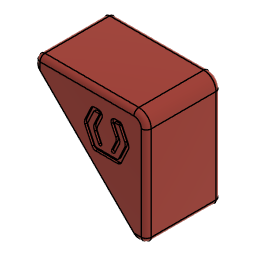
LogoRahmen (Autodesk Fusion 360 design; units mm, degrees)
Autodesk Fusion 360 part; units mm, degrees
box "Grundkörper Quader1" add length 240 width 240 height 3.2 placed x (0, 0, 1) y (1, 0, 0) z (0, 1, 0) at (0, 0, 0) makes body 1 in component "Canvas"
sketch "Skizze10" plane through (0, 0, 0) normal (0, -1, 0) x (1, 0, 0)
  line L0 (240, 240) -> (0, 240)
  line L1 (0, 240) -> (0, 0)
  line L2 (0, 0) -> (240, 0)
  line L3 (240, 0) -> (240, 240)
  line L4 (240, 0) -> (240, 240)
  line L5 (240, -11) -> (0, -11)
  line L6 (0, -11) -> (0, 8)
  line L7 (0, 8) -> (240, 8)
  line L8 (240, 8) -> (240, -11)
  line L9 (240, 120) -> (0, 120) construction
  line L10 (120, 240) -> (120, 0) construction
  line L11 (0, 251) -> (0, 232)
  line L12 (240, 251) -> (0, 251)
  line L13 (240, 232) -> (240, 251)
  line L14 (0, 232) -> (240, 232)
  line L15 (8, 232) -> (-11, 232)
  line L16 (-11, 232) -> (-11, 8)
  line L17 (-11, 8) -> (8, 8)
  line L18 (8, 8) -> (8, 232)
  line L19 (232, 8) -> (232, 232)
  line L20 (251, 232) -> (251, 8)
  line L21 (251, 8) -> (232, 8)
  line L22 (232, 232) -> (251, 232)
  dimension "d100" = 19
  dimension "d101" = 8
  dimension "d102" = 19
  dimension "d103" = 8
  constraint horizontal L5
  constraint vertical L6
  constraint horizontal L7
  constraint vertical L8
  constraint coincident L1 L6.end
  constraint collinear L4 L8
  constraint midpoint L3 L9.start
  constraint midpoint L1 L9.end
  constraint midpoint L0 L10.start
  constraint midpoint L2 L10.end
  constraint symmetric L5.start L9 L12.start
  constraint symmetric L5.end L9 L11.start
  constraint symmetric L6.end L9 L11.end
  constraint symmetric L7.end L9 L13.start
  constraint horizontal L15
  constraint vertical L16
  constraint horizontal L17
  constraint vertical L18
  constraint collinear L7 L17
  constraint collinear L14 L15
  constraint symmetric L10 L15.start L19.end
  constraint symmetric L10 L15.end L20.start
  constraint symmetric L10 L16.end L20.end
  constraint symmetric L10 L17.end L19.start
  measures "d100" distance of L5 L7
  measures "d101" distance of L2 L7
  measures "d102" distance of L16 L18
  measures "d103" distance of L1 L18
sketch "Skizze11" plane through (0, 3.2, 0) normal (0, 1, 0) x (-1, 0, 0)
  line L0 (0, 240) -> (-240, 240)
  line L1 (-240, 240) -> (-240, 0)
  line L2 (-240, 0) -> (0, 0)
  line L3 (0, 0) -> (0, 240)
  line L4 (-254, 254) -> (-209, 254)
  line L5 (-209, 254) -> (-209, 209)
  line L6 (-209, 209) -> (-254, 209)
  line L7 (-254, 209) -> (-254, 254)
  line L8 (-240, 251) -> (0, 251)
  line L9 (-251, 232) -> (-251, 8)
  line L10 (-209, 251) -> (-240, 251)
  line L11 (-251, 232) -> (-251, 209)
  line L12 (-251, 232) -> (-240, 232)
  line L13 (-240, 232) -> (-240, 251)
  line L14 (-240, 240) -> (-209, 240)
  line L15 (-240, 232) -> (-240, 209)
  dimension "d104" = 3
  dimension "d105" = 3
  dimension "d106" = 45
  dimension "d107" = 45
  constraint horizontal L4
  constraint vertical L5
  constraint horizontal L6
  constraint vertical L7
  constraint coincident L5 L10.start
  constraint coincident L8 L10.start
  constraint coincident L8.start L10.end
  constraint coincident L9.start L11.start
  constraint coincident L6 L11.end
  constraint coincident L9 L11.end
  constraint coincident L1 L12.end
  constraint perpendicular L1 L12
  constraint coincident L0.end L1.start
  constraint coincident L5 L14.end
  constraint coincident L0 L14.end
  constraint coincident L6 L15.end
  constraint coincident L1 L15.end
  measures "d104" distance of L4 L8
  measures "d105" distance of L7 L9
  measures "d106" distance of L5 L7
  measures "d107" distance of L4 L6
extrude "Extrusion1" add sketch "Skizze10" along normal blind 5 separate body contours L0 L1 L3 L4 L11 L13 L14 L15 L22 | L0 L11 L12 L13 makes body 2 in component "Rahmen"
extrude "Extrusion2" add sketch "Skizze10" along normal blind 5 separate body contours L3 L4 L20 L21 L22 | L3 L4 L7 L14 L19 L21 L22 makes body 3 in component "Rahmen"
extrude "Extrusion3" add sketch "Skizze10" along normal blind 5 separate body contours L1 L2 L3 L4 L6 L7 L8 L17 L21 | L2 L5 L6 L8 makes body 4 in component "Rahmen"
extrude "Extrusion4" add sketch "Skizze10" along normal blind 5 separate body contours L1 L7 L14 L15 L17 L18 | L1 L15 L16 L17 makes body 5 in component "Rahmen"
extrude "Extrusion1'" add sketch "Skizze11" along normal blind 27 from surface at -8 separate body contours L1 L4 L5 L6 L7 L8 L9 L10 L11 L12 L13 makes body 6 in component "Ecke"
sketch "Skizze1" plane through (0, -4.8, 0) normal (0, -1, 0) x (1, 0, 0) in component "Ecke"
  line L0 (240, 232) -> (251, 232)
  line L1 (251, 232) -> (251, 209)
  line L2 (251, 209) -> (254, 209)
  line L3 (254, 209) -> (254, 254)
  line L4 (254, 254) -> (209, 254)
  line L5 (209, 254) -> (209, 251)
  line L6 (209, 251) -> (240, 251)
  line L7 (240, 251) -> (240, 232)
  line L8 (251, 209) -> (209, 251)
  line L9 (209, 254) -> (254, 254)
  line L10 (254, 209) -> (254, 254)
  line L11 (251, 209) -> (254, 209)
  line L12 (209, 251) -> (209, 254)
  constraint coincident L1.end L2.start
  constraint coincident L5.end L6.start
  constraint coincident L4.end L5.start
  constraint coincident L3.end L4.start
  constraint coincident L2.end L3.start
extrude "Extrusion2'" add sketch "Skizze1" along normal blind 3.2 bodies 6 in component "Ecke"
copy_body "Körper kopieren/einfügen1" bodies 2 makes body 7 in component "Rahmen"
move_body "Verschieben1" bodies 7 to x (1, 0, 0) y (0, 0, 1) z (0, -1, 0) at (0, 251, 251) in component "Rahmen"
copy_body "Körper kopieren/einfügen2" bodies 3 makes body 8 in component "Rahmen"
move_body "Verschieben2" bodies 8 to x (0, -1, 0) y (1, 0, 0) z (0, 0, 1) at (251, 251, 0) in component "Rahmen"
extrude "Extrusion3'" add 1 faces at (229.6667, -4.8, 244.6667) along direction (0, 1, 0) blind 27 on bodies 6 bodies 6 in component "Ecke"
combine "Kombinieren1" operation cut target body 6 tool bodies 1 2 3 4 5 7 8 keep tools in component "Ecke"
move_face "Flächen versetzen1" offset -0.1 4 faces at (225.6667, -5, 244.6667) (219.3333, 11, 251) (251, 11, 224.3333) (233.3333, 3.2, 233.3333) on bodies 6 in component "Ecke"
sketch "Skizze2" plane through (0, 22.2, 0) normal (0, 1, 0) x (-1, 0, 0) in component "Ecke"
  line L0 (-251, 209) -> (-209, 251)
  line L1 (-209, 254) -> (-254, 254)
  line L2 (-254, 254) -> (-254, 209)
  line L3 (-230, 230) -> (-254, 254) construction
  line L4 (-240, 240) -> (-209, 240)
  line L5 (-240, 232) -> (-240, 209)
  line L6 (-240, 232) -> (-240, 251)
  line L7 (-209, 251) -> (-209, 254)
  line L8 (-254, 209) -> (-251, 209)
  point P0 (-234.5962, 234.5962)
  dimension "d144" = 6.5
  constraint midpoint L0 L3.start
  constraint coincident L1.end L2.start
  constraint coincident L3 P0
  measures "d144" distance of L0 P0
hole "Bohrung1" [suppressed] in component "Canvas"
hole "Bohrung3" at (234.5962, 22.2, 234.5962) direction (0, -1, 0) diameter 3.5 depth 21 tip angle 118 countersink diameter 7.5 countersink angle 90 bodies 6 in component "Ecke"
fillet "Abrundung1" radius 2 2 edges at (254, 7.1, 209) (209, 7.1, 254) on bodies 6 in component "Ecke"
fillet "Abrundung1" radius 5 1 edges at (254, 7.1, 254) on bodies 6 in component "Ecke"
fillet "Abrundung2" radius 2 14 edges at (251.5, -8, 209) (253.4142, -8, 209.5858) (254, -8, 230) (252.5355, -8, 252.5355) (230, -8, 254) (209.5858, -8, 253.4142) (209, -8, 251.5) (209, 22.2, 251.5) (209.5858, 22.2, 253.4142) (230, 22.2, 254) (252.5355, 22.2, 252.5355) (254, 22.2, 230) (253.4142, 22.2, 209.5858) (251.5, 22.2, 209) on bodies 6 in component "Ecke"
sketch "Skizze1 (2)" plane through (0, 0, 0) normal (0, 0, 1) x (1, 0, 0) in component "Logo v2"
  line L0 (6.3071, 6.0899) -> (0.8452, 8.6368)
  line L1 (-6.1226, 4.7416) -> (-0.1508, 7.5263)
  arc A0 (5.7, -4.99) -> (5.469, -5.3525) centre (5.3, -4.99) cw
  arc A1 (-0.1508, 7.5263) -> (0.1508, 7.5263) centre (0, 7.203) cw
  line L2 (-4.9747, -3.3762) -> (-0.8452, -5.3018)
  line L3 (-0.8452, -7.5086) -> (-6.1226, -5.0477)
  arc A2 (-6.7, 3.8352) -> (-6.1226, 4.7416) centre (-5.7, 3.8352) cw
  line L4 (0.8452, -5.3018) -> (5.4155, -3.1707)
  line L5 (7, 3.2028) -> (7, 5.0023)
  arc A3 (5.7, 3.0458) -> (5.4155, 2.8645) centre (5.5, 3.0458) cw
  arc A4 (-6.1226, -5.0477) -> (-6.7, -4.1414) centre (-5.7, -4.1414) cw
  line L6 (-4.4253, 1.8919) -> (-0.8, 3.5824)
  line L7 (-0.8452, 8.6368) -> (-7.0762, 5.7313)
  arc A5 (0.8452, 8.6368) -> (-0.8452, 8.6368) centre (0, 6.8242) ccw
  line L8 (5.469, -5.3525) -> (0.8452, -7.5086)
  arc A6 (5.469, 5.0463) -> (5.7, 4.6838) centre (5.3, 4.6838) cw
  arc A7 (4.7238, 1.7527) -> (7, 3.2028) centre (5.4, 3.2028) ccw
  arc A8 (-4.9747, 3.0701) -> (-4.4253, 1.8919) centre (-4.7, 2.481) ccw
  line L9 (0.8, 3.5824) -> (4.7238, 1.7527)
  line L10 (-1.3494, 4.7606) -> (-4.9747, 3.0701)
  line L11 (-6.7, -4.1414) -> (-6.7, 3.8352)
  arc A9 (1.3494, 4.7606) -> (-1.3494, 4.7606) centre (0, 1.8668) ccw
  line L12 (5.7, 4.6838) -> (5.7, 3.0458)
  arc A10 (7, 5.0023) -> (6.3071, 6.0899) centre (5.8, 5.0023) ccw
  arc A11 (-0.8, 3.5824) -> (0.8, 3.5824) centre (0, 1.8668) cw
  line L13 (5.7, -3.352) -> (5.7, -4.99)
  line L14 (-8, 4.2812) -> (-8, -4.5874)
  line L15 (4.7238, -2.0588) -> (0.8452, -3.8675)
  arc A12 (-4.4253, -2.198) -> (-4.9747, -3.3762) centre (-4.7, -2.7871) ccw
  line L16 (0.8452, -8.943) -> (6.3071, -6.3961)
  arc A13 (0.8452, -3.8675) -> (-0.8452, -3.8675) centre (0, -2.0548) cw
  arc A14 (7, -3.5089) -> (4.7238, -2.0588) centre (5.4, -3.5089) ccw
  line L17 (0.1508, 7.5263) -> (5.469, 5.0463)
  arc A15 (0.8452, -7.5086) -> (-0.8452, -7.5086) centre (0, -5.696) cw
  line L18 (-7.0762, -6.0375) -> (-0.8452, -8.943)
  arc A16 (-8, -4.5874) -> (-7.0762, -6.0375) centre (-6.4, -4.5874) ccw
  arc A17 (-0.8452, -8.943) -> (0.8452, -8.943) centre (0, -7.1304) ccw
  arc A18 (6.3071, -6.3961) -> (7, -5.3085) centre (5.8, -5.3085) ccw
  arc A19 (-0.8452, -5.3018) -> (0.8452, -5.3018) centre (0, -3.4892) ccw
  arc A20 (-7.0762, 5.7313) -> (-8, 4.2812) centre (-6.4, 4.2812) ccw
  line L19 (7, -5.3085) -> (7, -3.5089)
  arc A21 (5.4155, -3.1707) -> (5.7, -3.352) centre (5.5, -3.352) cw
  line L20 (5.4155, 2.8645) -> (1.3494, 4.7606)
  line L21 (-0.8452, -3.8675) -> (-4.4253, -2.198)
  line L22 (0, -9.1304) -> (0, 8.8242) construction
  constraint midpoint A17 L22.start
  constraint midpoint A5 L22.end
  constraint vertical L22
extrude "Extrusion1''" [suppressed] in component "Logo v2"
extrude "Extrusion5" cut sketch "Skizze1 (2)" against normal blind 1 sketch seen with x (0, 0, 1) y (-1, 0, 0) z (0, -1, 0) at (237.8129, -8.2, 240.0714) bodies 6 in component "Ecke"
component "Canvas" placed x (1, 0, 0) y (0, 1, 0) z (0, 0, 1) at (0, 0, 0)
component "Rahmen" placed x (1, 0, 0) y (0, 1, 0) z (0, 0, 1) at (0, 0, 0)
component "Ecke" placed x (1, 0, 0) y (0, 1, 0) z (0, 0, 1) at (0, 0, 0)
component "Logo v2" placed x (0, 0, 1) y (-1, 0, 0) z (0, -1, 0) at (237.8129, -8.2, 240.0714) in component "Ecke"
named bodies: "LogoRahmenEcke"
